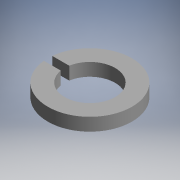
# Autodesk Inventor part: HCBST5_w1
Saved by Autodesk Inventor 2017.3 (Build 213256000, 256)
## iProperties
Part Number: HCBST5_w1
Material: Generic
Catalog Web Link: www.cadenas.de
Description: HCBST_washer1-Spring Washer Assembled Hexagon Socket Head Cap Screws
Vendor: MISUMI
Document SubType Name: Modeling
Designer: partserver
Manufacturer: MISUMI
Mass: 0.0453281 g
Surface Area: 1.27519 cm^2
Volume: 0.0453281 cm^3
Density: 1 g/cm^3
Appearance: PSOLRGB-192-192-192
Category: PARTsolutions
Company: MISUMI
Title: HCBST5
Author: Cadenas PARTsolutions
Comments: Spring Washer Assembled Hexagon Socket Head Cap Screws
PSOL_IDENT_0: {$CADENAS_DATA\23d-libs\misumi\metric\38_al_extrusions_blackets\nuts\hcbst_washer1.prj},162 {VTYP=3D
PSOL_IDENT_1: },{NB=HCBST5_w1},{LINA=HCBST5},{NN=HCBST_washer1},{DATE=18.04.2019 04:44:37},{GEOMDATE=15.04.2019 02
PSOL_IDENT_2: :23:09},{VERSION=},{LINEID=40},{WBVAR=},{WBNUMERIC=}  {NB=HCBST5_w1},{LINA=HCBST5},{KT=DUMMY},{PN=HC
PSOL_IDENT_3: BST5},{M=5},{M1=5},{MP=5x0.8},{P=0.800},{C=8.5},{D=10.0},{AA=5.4},{DD=5.1},{TT=1.3}
NB: HCBST5_w1
NN: HCBST_washer1
NT: Spring Washer Assembled Hexagon Socket Head Cap Screws
NBSYN: $PN._w1
LINA: HCBST5
CATALOG: Misumi
PN: HCBST5
M: 5
M1: 5
MP: 5x0.8
P: 0.8
C: 8.5
D: 10
AA: 5.4
DD: 5.1
TT: 1.3
SUPPLIER: MISUMI
ARTICLENO: HCBST5_w1
BOMINFO: HCBST5
CREATOR: CADENAS GmbH
Autodesk Inventor part; units mm, degrees
ref_plane "YZ Plane" through (0, 0, 0) normal (1, 0, 0) x (0, 1, 0)
ref_plane "XZ Plane" through (0, 0, 0) normal (0, 1, 0) x (-1, 0, 0)
ref_plane "XY Plane" through (0, 0, 0) normal (0, 0, 1) x (1, 0, 0)
sketch "Sketch_1" plane through (0, 0, 0) normal (0, 0, 1) x (1, 0, 0)
  arc A0 (4.2287, 0.425) -> (4.2287, -0.425) centre (0, 0) ccw
  line L0 (4.2287, -0.425) -> (2.5143, -0.425)
  arc A1 (2.5143, 0.425) -> (2.5143, -0.425) centre (0, 0) ccw
  line L1 (2.5143, 0.425) -> (4.2287, 0.425)
  constraints: 4 end point, 4 point on circle, 2 centre point
extrude "Extrusion1" add sketch "Sketch_1" against normal blind 1.3
ref_plane "spring_washer_to_bolt_XY" through (0, 0, 0) normal (0, 0, 1) x (1, 0, 0)
ref_plane "spring_washer_to_bolt_YZ" through (0, 0, 0) normal (1, 0, 0) x (0, 1, 0)
ref_plane "spring_washer_to_bolt_ZX" through (0, 0, 0) normal (0, 1, 0) x (0, 0, 1)
ref_plane "spring_washer_to_washer_XY" through (0, 0, -1.3) normal (0, 0, 1) x (1, 0, 0)
ref_plane "spring_washer_to_washer_YZ" through (0, 0, -1.3) normal (1, 0, 0) x (0, 1, 0)
ref_plane "spring_washer_to_washer_ZX" through (0, 0, -1.3) normal (0, 1, 0) x (0, 0, 1)
body "Solid1"
